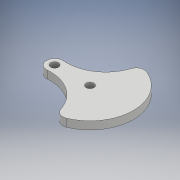
# Autodesk Inventor part: кривошип_v3
Saved by Autodesk Inventor 2017.3 (Build 213256000, 256)
## iProperties
Part Number: кривошип_v3
Material: Типовые
Document SubType Name: Modeling
Designer: Alexnav
Density: 1 g/cm^3
Appearance: По умолчанию
Author: Alexnav
Autodesk Inventor part; units mm, degrees
ref_plane "YZ Plane" through (0, 0, 0) normal (1, 0, 0) x (0, 1, 0)
ref_plane "XZ Plane" through (0, 0, 0) normal (0, 1, 0) x (-1, 0, 0)
ref_plane "XY Plane" through (0, 0, 0) normal (0, 0, 1) x (1, 0, 0)
sketch "Эскиз1" plane through (0, 0, 0) normal (0, 0, 1) x (1, 0, 0)
  circle A0 centre (0, 0) radius 5
  circle A1 centre (0, 0) radius 55
  dimension "d0" = 10
  dimension "d1" = 110
  constraints: 2 centre point, 2 coincident
  measures "d0" diameter of A0
  measures "d1" diameter of A1
extrude "Выдавливание1" add sketch "Эскиз1" along normal blind 10
sketch "Эскиз2" plane through (0, 0, 10) normal (0, 0, 1) x (1, 0, 0)
  circle A0 centre (-40, 60) radius 50
  line L0 (0, -92.4934) -> (0, 92.4934) projected
  line L1 (-90.2801, 0) -> (79.2133, 0) projected
  circle A1 centre (-40, -60) radius 50
  point P0 (0, 0)
  dimension "d4" = 60
  dimension "d5" = 40
  dimension "d14" = 100
  constraints: 2 centre point, 1 equal radius, 1 other
  measures "d4" distance from line of A0.centre L1
  measures "d5" distance from line of L0 A0.centre
  measures "d14" diameter of A0
extrude "Выдавливание2" cut sketch "Эскиз2" against normal through all
fillet "Сопряжение1" radius 10 2 edges at (-53.6946, 11.912, 5) (-53.6946, -11.912, 5)
fillet "Сопряжение2" radius 10 2 edges at (9.6561, 54.1457, 5) (9.6561, -54.1457, 5)
sketch "Эскиз3" plane through (0, 0, 10) normal (0, 0, 1) x (1, 0, 0)
  circle A0 centre (0, 0) radius 5 projected
  line L0 (-77, 0) -> (77, 0) projected
  circle A1 centre (-45, 0) radius 5
  dimension "d10" = 10
  dimension "d11" = 45
  constraints: 1 centre point, 1 point on line
  measures "d10" diameter of A1
  measures "d11" distance of point (0, 0) A1.centre
extrude "Выдавливание3" cut sketch "Эскиз3" against normal through all contours A1 L0 | L0 A1
